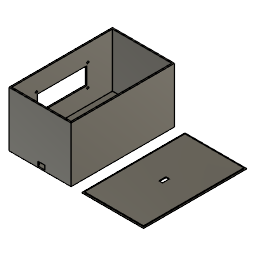
Station Météo (Autodesk Fusion 360 design; units mm, degrees)
part number: 2026-03-28-17-40-34-865
Autodesk Fusion 360 part; units mm, degrees
sketch "Esquisse1" plane through (0, 0, 0) normal (0, 0, 1) x (1, 0, 0)
  line L0 (0, 0) -> (90, 0)
  line L1 (90, 0) -> (90, 150)
  line L2 (90, 150) -> (0, 150)
  line L3 (0, 150) -> (0, 0)
  dimension "d42" = 90
  dimension "d43" = 150
  constraint horizontal L0
  constraint vertical L1
  constraint horizontal L2
  constraint vertical L3
  constraint coincident L0.start L3.end
  measures "d42" distance of L0.start L0.end
  measures "d43" distance of L0.start L2.end
extrude "Extrusion1" add sketch "Esquisse1" along normal blind 80 makes body 1
shell "Coque1" thickness 2 removed faces 1 at (30, 100, 80) on bodies 1
sketch "Esquisse2" plane through (0, 0, 0) normal (-1, 0, 0) x (0, -1, 0)
  line L0 (-150, 0) -> (0, 0)
  line L1 (0, 0) -> (0, 80)
  line L2 (0, 80) -> (-150, 80)
  line L3 (-150, 80) -> (-150, 0)
  line L4 (-110.7, 52.5) -> (-39.3, 52.5)
  line L5 (-39.3, 52.5) -> (-39.3, 27.5)
  line L6 (-39.3, 27.5) -> (-110.7, 27.5)
  line L7 (-110.7, 27.5) -> (-110.7, 52.5)
  line L8 (-150, 40) -> (-110.7, 40) construction
  line L9 (-39.3, 40) -> (0, 40) construction
  line L10 (-112.25, 24) -> (-37.75, 24) construction
  line L11 (-37.75, 24) -> (-37.75, 56) construction
  line L12 (-37.75, 56) -> (-112.25, 56) construction
  line L13 (-112.25, 56) -> (-112.25, 24) construction
  line L14 (-75, 56) -> (-75, 80)
  line L15 (-75, 24) -> (-75, 0)
  dimension "d32" = 25
  dimension "d33" = 71.4
  dimension "d40" = 1.55
  dimension "d41" = 3.5
  constraint horizontal L4
  constraint vertical L5
  constraint horizontal L6
  constraint vertical L7
  constraint midpoint L3 L8.start
  constraint midpoint L7 L8.end
  constraint midpoint L5 L9.start
  constraint midpoint L1 L9.end
  constraint equal L8 L9
  constraint horizontal L8
  constraint horizontal L10
  constraint vertical L11
  constraint horizontal L12
  constraint vertical L13
  constraint midpoint L12 L14.start
  constraint midpoint L2 L14.end
  constraint midpoint L10 L15.start
  constraint midpoint L0 L15.end
  constraint equal L14 L15
  constraint vertical L14
  measures "d32" distance of L4.end L5.end
  measures "d33" distance of L4.start L4.end
  measures "d40" distance of L7 L13
  measures "d41" distance of L6 L10
extrude "Extrusion2" cut sketch "Esquisse2" against normal blind 10 contours L4 L5 L6 L7 bodies 1
sketch "Esquisse6" plane through (0, 0, 0) normal (0, -1, 0) x (1, 0, 0)
  line L0 (0, 0) -> (90, 0)
  line L1 (90, 0) -> (90, 80)
  line L2 (90, 80) -> (0, 80)
  line L3 (0, 80) -> (0, 0)
  line L4 (42, 2) -> (52, 2)
  line L5 (52, 2) -> (52, 8)
  line L6 (52, 8) -> (42, 8)
  line L7 (42, 8) -> (42, 2)
  constraint horizontal L4
  constraint vertical L5
  constraint horizontal L6
  constraint vertical L7
extrude "Extrusion5" cut sketch "Esquisse6" against normal blind 2 contours L4 L5 L6 L7 bodies 1
sketch "Esquisse9" plane through (0, 0, 0) normal (0, 0, 1) x (1, 0, 0)
  line L0 (105, 0) -> (195, 0)
  line L1 (195, 0) -> (195, 150)
  line L2 (195, 150) -> (105, 150)
  line L3 (105, 150) -> (105, 0)
  line L4 (192.8, 147.8) -> (107.2, 147.8)
  line L5 (107.2, 147.8) -> (107.2, 2.2)
  line L6 (107.2, 2.2) -> (192.8, 2.2)
  line L7 (192.8, 2.2) -> (192.8, 147.8)
  line L8 (0, 0) -> (90, 0)
  line L9 (90, 150) -> (0, 150)
  dimension "d34" = -2.2
  dimension "d35" = 15
  constraint horizontal L0
  constraint vertical L1
  constraint horizontal L2
  constraint vertical L3
  constraint collinear L0 L8
  constraint collinear L2 L9
  constraint equal L0 L8
  measures "d35" distance of L3 L9.start
extrude "Extrusion9" add sketch "Esquisse9" along normal blind 0.2 separate body contours L0 L1 L2 L3 | L4 L5 L6 L7 makes body 2
extrude "Extrusion10" add sketch "Esquisse9" along normal blind 1.2 contours L4 L5 L6 L7 bodies 2
sketch "Esquisse11" plane through (0, 0, 1.2) normal (0, 0, 1) x (-1, 0, 0)
  line L0 (-152.5, -70) -> (-147.5, -70)
  line L1 (-147.5, -70) -> (-147.5, -80)
  line L2 (-147.5, -80) -> (-152.5, -80)
  line L3 (-152.5, -80) -> (-152.5, -70)
  line L4 (-192.8, -2.2) -> (-192.8, -147.8)
  line L5 (-192.8, -147.8) -> (-107.2, -147.8)
  line L6 (-107.2, -147.8) -> (-107.2, -2.2)
  line L7 (-107.2, -2.2) -> (-192.8, -2.2)
  line L8 (-192.8, -2.2) -> (-192.8, -147.8)
  line L9 (-107.2, -147.8) -> (-107.2, -2.2)
  line L10 (-150, -70) -> (-150, -2.2) construction
  line L11 (-150, -80) -> (-150, -147.8) construction
  line L12 (-192.8, -75) -> (-152.5, -75) construction
  line L13 (-147.5, -75) -> (-107.2, -75) construction
  dimension "d28" = 5
  dimension "d29" = 10
  constraint horizontal L0
  constraint vertical L1
  constraint horizontal L2
  constraint vertical L3
  constraint midpoint L0 L10.start
  constraint midpoint L7 L10.end
  constraint midpoint L2 L11.start
  constraint midpoint L5 L11.end
  constraint equal L10 L11
  constraint midpoint L4 L12.start
  constraint midpoint L3 L12.end
  constraint midpoint L1 L13.start
  constraint midpoint L6 L13.end
  constraint equal L12 L13
  measures "d28" distance of L0.start L0.end
  measures "d29" distance of L0.end L1.end
extrude "Extrusion11" cut sketch "Esquisse11" against normal up to surface (1.2 mm away) contours L0 L1 L2 L3 bodies 2
hole "Perçage2" at (0, 112.25, 56) at (0, 37.75, 56) at (0, 37.75, 24) at (0, 112.25, 24) direction (1, 0, 0) diameter 3 depth 3 tip angle 118 bodies 1
equation "d26 = 0.2 mm + 1 mm"
equation "d40 = 4.25 mm - 2.5 mm - 0.2 mm"
equation "d41 = 6 mm - 2.5 mm"
